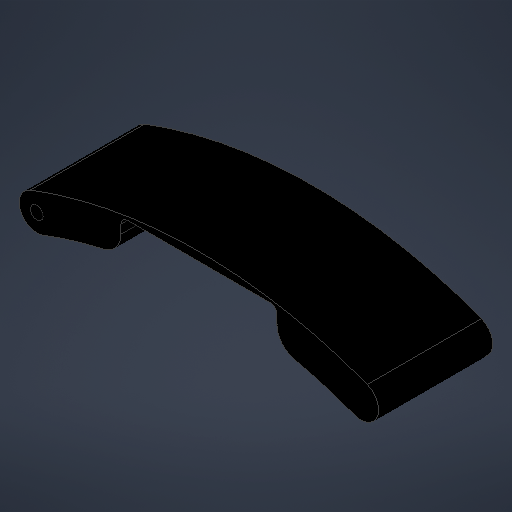
# Autodesk Inventor part: Part2
Saved by Autodesk Inventor 2026.1 (Build 301233020, 233B)
## iProperties
Created: 2026-02-15
Part Number: Part2
Material: Generic
Document SubType Name: Modeling
Designer: Bahaa
Density: 1 g/cm^3
Appearance: Default
Author: Bahaa
Autodesk Inventor part; units mm, degrees
ref_plane "YZ Plane" through (0, 0, 0) normal (1, 0, 0) x (0, 1, 0)
ref_plane "XZ Plane" through (0, 0, 0) normal (0, 1, 0) x (-1, 0, 0)
ref_plane "XY Plane" through (0, 0, 0) normal (0, 0, 1) x (1, 0, 0)
derived "Bottom Ring.ipt"
sketch "Sketch9" plane through (0, 4, 0) normal (0, 1, 0) x (1, 0, 0)
  circle A0 centre (-36.9121, -96.6941) radius 1.6 projected
  circle A1 centre (-36.9121, -96.6941) radius 4 projected
  arc A2 (-38.154, -91.8941) -> (-20.75, -97.3123) centre (0, 0) ccw projected
  circle A3 centre (-36.9121, -96.6941) radius 1.6 projected
  line L0 (-38.154, -91.8941) -> (-44.2364, -97.9765) projected
  arc A4 (-44.2364, -97.9765) -> (44.2364, -97.9765) centre (0, 0) ccw projected
  line L1 (44.2364, -97.9765) -> (38.154, -91.8941) projected
  arc A5 (20.75, -97.3123) -> (38.154, -91.8941) centre (0, 0) ccw projected
  arc A6 (17.75, -97.904) -> (20.75, -97.3123) centre (0, 0) ccw projected
  line L2 (17.75, -97.904) -> (17.75, -104) projected
  arc A7 (16.25, -105.5) -> (17.75, -104) centre (16.25, -104) ccw projected
  line L3 (16.25, -105.5) -> (-16.25, -105.5) projected
  arc A8 (-17.75, -104) -> (-16.25, -105.5) centre (-16.25, -104) ccw projected
  line L4 (-17.75, -104) -> (-17.75, -97.904) projected
  arc A9 (-20.75, -97.3123) -> (-17.75, -97.904) centre (0, 0) ccw projected
  arc A10 (-38.154, -91.8941) -> (-20.75, -97.3123) centre (0, 0) ccw projected
  line L5 (0, -107.5) -> (0, -105.5) construction
  circle A11 centre (36.9121, -96.6941) radius 4 projected
  circle A12 centre (-36.9121, -96.6941) radius 1.45
  point P0 (-35.4855, -92.9571)
  point P1 (-38.3387, -100.4311)
  point P2 (38.3387, -100.4311)
  point P3 (35.4855, -92.9571)
  point P4 (-20.75, -97.3123)
  dimension "d4" = 0.15
  constraints: 1 centre point
  measures "d4" radial gap between concentric circles of A0 A12
extrude "Extrusion1" add sketch "Sketch9" along normal blind 26 contours A0 | A1 | A1 A2 A9 L4 A8 L3 A7 L2 A6 A5 A11 A4 | A11 | A12
fillet "Fillet1" radius 5 2 edges at (17.75, 17, 97.904) (-17.75, 17, 97.904)
extrude "Extrusion2" cut sketch "Sketch9" along normal blind 21 contours A12
sketch "Sketch2" plane through (0, 30, 0) normal (0, 1, 0) x (1, 0, 0)
  point P0 (0, 0)
  point P1 (36.9121, -96.6941)
hole "Hole1" at (36.9121, 30, 96.6941) direction (0, -1, 0) diameter 4.2 depth 6
body "Solid1"
